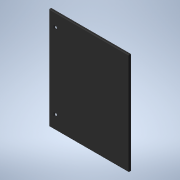
# Autodesk Inventor part: 1676X_01_01(1)_P2
Saved by Autodesk Inventor 2021 (Build 250183000, 183)
## iProperties
Created: 2025-05-05
Part Number: 1676X_01_01(1)_P2
Material: Generic
Catalog Web Link: www.cadenas.de
Description: AE 2.0 Einzeltuer-AE 2.0 Einzeltuer
Vendor: RITTAL
Document SubType Name: Modeling
Designer: psAdmin
Manufacturer: RITTAL
Mass: 1137.32 g
Surface Area: 10932.5 cm^2
Volume: 1137.32 cm^3
Density: 1 g/cm^3
Appearance: PSOLRGB-175-175-175
Category: PARTsolutions
Company: RITTAL
Title: 1676X_01_01(1)_P2
Author: Cadenas PARTsolutions
Comments: AE 2.0 Einzeltuer
PSOL_IDENT_0: {$CADENAS_DATA/23d-libs/rittal/schaltschranksys/kompakt_schaltschr/parts_ae_2_0/einzeltuer_ae_2_0.pr
PSOL_IDENT_1: j},198 {VTYP=3D},{NB=1676X_01_01(1)_P2},{LINA=1676X_01_01(1)_P2},{NN=AE 2.0 Einzeltuer},{DATE=28.04.
PSOL_IDENT_2: 2025 21:11:31},{GEOMDATE=11.04.2025 11:21:47},{VERSION=},{LINEID=330},{WBVAR=DETAIL},{WBNUMERIC=DETA
PSOL_IDENT_3: IL}  {NB=1676X_01_01(1)_P2},{LINA=1676X_01_01(1)_P2},{KT=DUMMY},{BEST=1676X},{DETAIL=1},{BEZ1=Neues
PSOL_IDENT_4: Kompaktgehäuse},{BEZ2=Stahlblech},{BEZ3=eintürig},{B=600},{H=760},{VERS=1},{W=595},{W1=525},{W3=0},{
PSOL_IDENT_5: HH=755},{H1=635},{H2=700},{H4=58.0},{H5=560.000},{H6=600.000},{H7=500.000},{D=15.0},{ST=2.0},{R1=5.0
PSOL_IDENT_6: },{GEW=0},{CNSECLASS51=27-18-01-02},{CNSECLASS70=27-18-01-01},{CNSECLASS80=27-18-01-01},{CNSETIM40=E
PSOL_IDENT_7: C000261}
NB: 1676X_01_01(1)_P2
NN: AE 2.0 Einzeltuer
NT: AE 2.0 Einzeltuer
NBSYN: $BEST._01_01($DETAIL.)_P2
LINA: 1676X_01_01(1)_P2
CATALOG: Rittal
BEST: 1676X
DETAIL: hoch
BEZ1: Neues Kompaktgehäuse
BEZ2: Stahlblech
BEZ3: eintürig
B: 600
H: 760
VERS: 1
W: 595
W1: 525
W3: 0
HH: 755
H1: 635
H2: 700
H4: 58
H5: 560
H6: 600
H7: 500
D: 15
ST: 2
R1: 5
GEW: 0
CNSECLASS70: 27-18-01-01
CNSECLASS80: 27-18-01-01
SUPPLIER: RITTAL
ARTICLENO: 1676X_01_01(1)_P2
BOMINFO: 1676X_01_01(1)_P2
CREATOR: CADENAS GmbH
Autodesk Inventor part; units mm, degrees
sketch "Sketch_1" plane through (0, 0, 0) normal (0, 1, 0) x (1, 0, 0)
  arc A0 (-297.5, 5) -> (-292.5, 0) centre (-292.5, 5) ccw
  line L0 (-292.5, 0) -> (292.5, 0)
  arc A1 (292.5, 0) -> (297.5, 5) centre (292.5, 5) ccw
  line L1 (297.5, 5) -> (297.5, 15)
  line L2 (297.5, 15) -> (295.5, 15)
  line L3 (295.5, 15) -> (295.5, 5)
  arc A2 (292.5, 2) -> (295.5, 5) centre (292.5, 5) ccw
  line L4 (292.5, 2) -> (-292.5, 2)
  arc A3 (-295.5, 5) -> (-292.5, 2) centre (-292.5, 5) ccw
  line L5 (-295.5, 5) -> (-295.5, 15)
  line L6 (-295.5, 15) -> (-297.5, 15)
  line L7 (-297.5, 15) -> (-297.5, 5)
  constraints: 16 end point, 8 point on circle, 4 centre point
extrude "Extrusion1" add sketch "Sketch_1" along normal mid plane 745
sketch "Sketch_3" plane through (0, 372.5, 0) normal (0, 1, 0) x (1, 0, 0)
  line L0 (292.5, 0) -> (292.5, 15)
  arc A0 (292.5, 2) -> (295.5, 5) centre (292.5, 5) ccw
  line L1 (295.5, 5) -> (295.5, 15)
  line L2 (295.5, 15) -> (297.5, 15)
  line L3 (297.5, 15) -> (297.5, 5)
  arc A1 (292.5, 0) -> (297.5, 5) centre (292.5, 5) ccw
  line L4 (292.5, 0) -> (292.5, 2)
  constraints: 10 end point, 4 point on circle, 2 centre point
revolve "Revolution1" add sketch "Sketch_3" angle 90 about axis through (292.5, 372.5, 0) along (0, 0, 1)
sketch "Sketch_4" plane through (0, 372.5, 0) normal (0, 1, 0) x (1, 0, 0)
  line L0 (-292.5, 15) -> (-292.5, 0)
  arc A0 (-297.5, 5) -> (-292.5, 0) centre (-292.5, 5) ccw
  line L1 (-297.5, 5) -> (-297.5, 15)
  line L2 (-297.5, 15) -> (-295.5, 15)
  line L3 (-295.5, 15) -> (-295.5, 5)
  arc A1 (-295.5, 5) -> (-292.5, 2) centre (-292.5, 5) ccw
  line L4 (-292.5, 2) -> (-292.5, 0)
  constraints: 10 end point, 4 point on circle, 2 centre point
revolve "Revolution2" add sketch "Sketch_4" angle 90 about axis through (-292.5, 372.5, -15) along (0, 0, -1)
sketch "Sketch_5" plane through (0, -372.5, 0) normal (0, 1, 0) x (1, 0, 0)
  line L0 (292.5, 0) -> (292.5, 15)
  arc A0 (292.5, 2) -> (295.5, 5) centre (292.5, 5) ccw
  line L1 (295.5, 5) -> (295.5, 15)
  line L2 (295.5, 15) -> (297.5, 15)
  line L3 (297.5, 15) -> (297.5, 5)
  arc A1 (292.5, 0) -> (297.5, 5) centre (292.5, 5) ccw
  line L4 (292.5, 0) -> (292.5, 2)
  constraints: 10 end point, 4 point on circle, 2 centre point
revolve "Revolution3" add sketch "Sketch_5" angle 90 about axis through (292.5, -372.5, 0) along (0, 0, -1)
sketch "Sketch_6" plane through (0, -372.5, 0) normal (0, 1, 0) x (1, 0, 0)
  line L0 (-292.5, 15) -> (-292.5, 0)
  arc A0 (-297.5, 5) -> (-292.5, 0) centre (-292.5, 5) ccw
  line L1 (-297.5, 5) -> (-297.5, 15)
  line L2 (-297.5, 15) -> (-295.5, 15)
  line L3 (-295.5, 15) -> (-295.5, 5)
  arc A1 (-295.5, 5) -> (-292.5, 2) centre (-292.5, 5) ccw
  line L4 (-292.5, 2) -> (-292.5, 0)
  constraints: 10 end point, 4 point on circle, 2 centre point
revolve "Revolution4" add sketch "Sketch_6" angle 90 about axis through (-292.5, -372.5, -15) along (0, 0, 1)
sketch "Sketch_2" plane through (0, 0, 0) normal (1, 0, 0) x (0, 0, -1)
  line L0 (0, 372.5) -> (0, -372.5)
  arc A0 (0, -372.5) -> (5, -377.5) centre (5, -372.5) ccw
  line L1 (5, -377.5) -> (15, -377.5)
  line L2 (15, -377.5) -> (15, -375.5)
  line L3 (15, -375.5) -> (5, -375.5)
  arc A1 (2, -372.5) -> (5, -375.5) centre (5, -372.5) ccw
  line L4 (2, -372.5) -> (2, 372.5)
  arc A2 (5, 375.5) -> (2, 372.5) centre (5, 372.5) ccw
  line L5 (5, 375.5) -> (15, 375.5)
  line L6 (15, 375.5) -> (15, 377.5)
  line L7 (15, 377.5) -> (5, 377.5)
  arc A3 (5, 377.5) -> (0, 372.5) centre (5, 372.5) ccw
  constraints: 16 end point, 8 point on circle, 4 centre point
extrude "Extrusion2" add sketch "Sketch_2" along normal mid plane 585
sketch "Sketch_44" plane through (281, 0, 0) normal (1, 0, 0) x (0, 0, -1)
  line L0 (2, -354.6934) -> (2, 354.6934)
  line L1 (2, 354.6934) -> (8, 354.6934)
  line L2 (8, 354.6934) -> (7.5, 338)
  line L3 (7.5, 338) -> (7.5, -338)
  line L4 (7.5, -338) -> (8, -354.6934)
  line L5 (8, -354.6934) -> (2, -354.6934)
  line L6 (2, -354.6934) -> (2, 354.6934)
  constraints: 14 end point
revolve "Revolution5" add sketch "Sketch_44" angle 180 mid plane about axis through (281, -354.6934, -2) along (0, 1, 0)
sketch "Sketch_45" plane through (0, 354.6934, 0) normal (0, 1, 0) x (1, 0, 0)
  line L0 (291, 8) -> (291, 2)
  line L1 (275, 2) -> (287, 2)
  arc A0 (287, 2) -> (275, 2) centre (281, 2) ccw
  constraints: 4 end point, 2 point on circle, 1 centre point
revolve "Revolution6" add sketch "Sketch_45" angle 39.715 about axis through (291, 354.6934, -8) along (0, 0, -1)
sketch "Sketch_47" plane through (0, 354.6934, 0) normal (0, 1, 0) x (1, 0, 0)
  line L0 (-291, 2) -> (-291, 8)
  line L1 (-287, 2) -> (-275, 2)
  arc A0 (-275, 2) -> (-287, 2) centre (-281, 2) ccw
  constraints: 4 end point, 2 point on circle, 1 centre point
revolve "Revolution7" add sketch "Sketch_47" angle 39.715 about axis through (-291, 354.6934, -2) along (0, 0, 1)
sketch "Sketch_46" plane through (291, 354.6934, 0) normal (-0.6389711, -0.7692308, 0) x (-0.7692308, 0.6389711, 0)
  line L0 (13, 7.1962) -> (13, 2)
  line L1 (13, 2) -> (4, 2)
  arc A0 (13, 7.1962) -> (4, 2) centre (10, 2) ccw
  line L2 (13, 7.1962) -> (13, 2)
  constraints: 6 end point, 2 point on circle, 1 centre point
revolve "Revolution8" add sketch "Sketch_46" angle 169.43 about axis through (281, 363, -7.1962) along (0, 0, 1)
sketch "Sketch_49" plane through (-291, 354.6934, 0) normal (-0.6389711, 0.7692308, 0) x (0.7692308, 0.6389711, 0)
  line L0 (13, 7.1962) -> (13, 2)
  line L1 (13, 2) -> (4, 2)
  arc A0 (13, 7.1962) -> (4, 2) centre (10, 2) ccw
  line L2 (13, 7.1962) -> (13, 2)
  constraints: 6 end point, 2 point on circle, 1 centre point
revolve "Revolution9" add sketch "Sketch_49" angle 169.43 about axis through (-281, 363, -7.1962) along (0, 0, -1)
sketch "Sketch_48" plane through (281, 363, 0) normal (-0.7692308, -0.6389711, 0) x (-0.6389711, 0.7692308, 0)
  line L0 (13, 8) -> (13, 2)
  line L1 (-3, 2) -> (9, 2)
  arc A0 (9, 2) -> (-3, 2) centre (3, 2) ccw
  constraints: 4 end point, 2 point on circle, 1 centre point
revolve "Revolution10" add sketch "Sketch_48" angle 39.715 about axis through (272.6934, 373, -8) along (0, 0, -1)
sketch "Sketch_50" plane through (-281, 363, 0) normal (-0.7692308, 0.6389711, 0) x (0.6389711, 0.7692308, 0)
  line L0 (13, 8) -> (13, 2)
  line L1 (-3, 2) -> (9, 2)
  arc A0 (9, 2) -> (-3, 2) centre (3, 2) ccw
  constraints: 4 end point, 2 point on circle, 1 centre point
revolve "Revolution11" add sketch "Sketch_50" angle 39.715 about axis through (-272.6934, 373, -8) along (0, 0, 1)
sketch "Sketch_51" plane through (-281, 0, 0) normal (1, 0, 0) x (0, 0, -1)
  line L0 (2, -354.6934) -> (2, 354.6934)
  line L1 (2, 354.6934) -> (8, 354.6934)
  line L2 (8, 354.6934) -> (7.5, 338)
  line L3 (7.5, 338) -> (7.5, -338)
  line L4 (7.5, -338) -> (8, -354.6934)
  line L5 (8, -354.6934) -> (2, -354.6934)
  line L6 (2, -354.6934) -> (2, 354.6934)
  constraints: 14 end point
revolve "Revolution12" add sketch "Sketch_51" angle 180 mid plane about axis through (-281, -354.6934, -2) along (0, 1, 0)
sketch "Sketch_52" plane through (0, -354.6934, 0) normal (0, 1, 0) x (1, 0, 0)
  line L0 (291, 8) -> (291, 2)
  line L1 (275, 2) -> (287, 2)
  arc A0 (287, 2) -> (275, 2) centre (281, 2) ccw
  constraints: 4 end point, 2 point on circle, 1 centre point
revolve "Revolution13" add sketch "Sketch_52" angle 39.715 about axis through (291, -354.6934, -8) along (0, 0, 1)
sketch "Sketch_53" plane through (0, -354.6934, 0) normal (0, 1, 0) x (1, 0, 0)
  line L0 (-291, 2) -> (-291, 8)
  line L1 (-287, 2) -> (-275, 2)
  arc A0 (-275, 2) -> (-287, 2) centre (-281, 2) ccw
  constraints: 4 end point, 2 point on circle, 1 centre point
revolve "Revolution14" add sketch "Sketch_53" angle 39.715 about axis through (-291, -354.6934, -2) along (0, 0, -1)
sketch "Sketch_54" plane through (291, -354.6934, 0) normal (0.6389711, -0.7692308, 0) x (-0.7692308, -0.6389711, 0)
  line L0 (13, 7.1962) -> (13, 2)
  line L1 (13, 2) -> (4, 2)
  arc A0 (13, 7.1962) -> (4, 2) centre (10, 2) ccw
  line L2 (13, 7.1962) -> (13, 2)
  constraints: 6 end point, 2 point on circle, 1 centre point
revolve "Revolution15" add sketch "Sketch_54" angle 169.43 about axis through (281, -363, -7.1962) along (0, 0, -1)
sketch "Sketch_55" plane through (281, -363, 0) normal (0.7692308, -0.6389711, 0) x (-0.6389711, -0.7692308, 0)
  line L0 (13, 8) -> (13, 2)
  line L1 (-3, 2) -> (9, 2)
  arc A0 (9, 2) -> (-3, 2) centre (3, 2) ccw
  constraints: 4 end point, 2 point on circle, 1 centre point
revolve "Revolution16" add sketch "Sketch_55" angle 39.715 about axis through (272.6934, -373, -8) along (0, 0, 1)
sketch "Sketch_56" plane through (-291, -354.6934, 0) normal (-0.6389711, -0.7692308, 0) x (-0.7692308, 0.6389711, 0)
  line L0 (-13, 2) -> (-13, 7.1962)
  arc A0 (-4, 2) -> (-13, 7.1962) centre (-10, 2) ccw
  line L1 (-4, 2) -> (-13, 2)
  line L2 (-13, 2) -> (-13, 7.1962)
  constraints: 6 end point, 2 point on circle, 1 centre point
revolve "Revolution17" add sketch "Sketch_56" angle 169.43 about axis through (-281, -363, -2) along (0, 0, 1)
sketch "Sketch_57" plane through (-281, -363, 0) normal (0.7692308, 0.6389711, 0) x (0.6389711, -0.7692308, 0)
  line L0 (13, 8) -> (13, 2)
  line L1 (-3, 2) -> (9, 2)
  arc A0 (9, 2) -> (-3, 2) centre (3, 2) ccw
  constraints: 4 end point, 2 point on circle, 1 centre point
revolve "Revolution18" add sketch "Sketch_57" angle 39.715 about axis through (-272.6934, -373, -8) along (0, 0, -1)
sketch "Sketch_58" plane through (0, 363, 0) normal (0, 1, 0) x (1, 0, 0)
  line L0 (272.6934, 2) -> (-272.6934, 2)
  line L1 (-272.6934, 2) -> (-272.6934, 8)
  line L2 (-272.6934, 8) -> (272.6934, 8)
  line L3 (272.6934, 8) -> (272.6934, 2)
  line L4 (272.6934, 2) -> (-272.6934, 2)
  constraints: 10 end point
revolve "Revolution19" add sketch "Sketch_58" angle 180 mid plane about axis through (272.6934, 363, -2) along (-1, 0, 0)
sketch "Sketch_59" plane through (0, -363, 0) normal (0, 1, 0) x (1, 0, 0)
  line L0 (272.6934, 2) -> (-272.6934, 2)
  line L1 (-272.6934, 2) -> (-272.6934, 8)
  line L2 (-272.6934, 8) -> (272.6934, 8)
  line L3 (272.6934, 8) -> (272.6934, 2)
  line L4 (272.6934, 2) -> (-272.6934, 2)
  constraints: 10 end point
revolve "Revolution20" add sketch "Sketch_59" angle 180 mid plane about axis through (272.6934, -363, -2) along (-1, 0, 0)
sketch "Sketch_7" plane through (0, -317.5, 0) normal (0, 1, 0) x (1, 0, 0)
  arc A0 (290.5, 15.1) -> (290.5, 6.9) centre (290.5, 11) ccw
  line L0 (290.5, 6.9) -> (295.5, 6.9)
  line L1 (295.5, 6.9) -> (295.5, 8.4)
  line L2 (295.5, 8.4) -> (290.5, 8.4)
  arc A1 (290.5, 13.6) -> (290.5, 8.4) centre (290.5, 11) ccw
  line L3 (290.5, 13.6) -> (295.5, 13.6)
  line L4 (295.5, 13.6) -> (295.5, 15.1)
  line L5 (295.5, 15.1) -> (290.5, 15.1)
  constraints: 12 end point, 4 point on circle, 2 centre point
extrude "Extrusion3" add sketch "Sketch_7" along normal mid plane 19.7
sketch "Sketch_8" plane through (0, 317.5, 0) normal (0, 1, 0) x (1, 0, 0)
  arc A0 (290.5, 15.1) -> (290.5, 6.9) centre (290.5, 11) ccw
  line L0 (290.5, 6.9) -> (295.5, 6.9)
  line L1 (295.5, 6.9) -> (295.5, 8.4)
  line L2 (295.5, 8.4) -> (290.5, 8.4)
  arc A1 (290.5, 13.6) -> (290.5, 8.4) centre (290.5, 11) ccw
  line L3 (290.5, 13.6) -> (295.5, 13.6)
  line L4 (295.5, 13.6) -> (295.5, 15.1)
  line L5 (295.5, 15.1) -> (290.5, 15.1)
  constraints: 12 end point, 4 point on circle, 2 centre point
extrude "Extrusion4" add sketch "Sketch_8" along normal mid plane 19.7
sketch "Sketch_11" plane through (0, 0, 0) normal (0, 1, 0) x (1, 0, 0)
  line L0 (254.5, 15.9) -> (254.5, 2)
  line L1 (254.5, 2) -> (255.3, 2)
  line L2 (255.3, 2) -> (255.3, 15.9)
  arc A0 (256.1, 16.7) -> (255.3, 15.9) centre (256.1, 15.9) ccw
  line L3 (256.1, 16.7) -> (268.4, 16.7)
  arc A1 (269.2, 15.9) -> (268.4, 16.7) centre (268.4, 15.9) ccw
  line L4 (269.2, 15.9) -> (269.2, 2)
  line L5 (269.2, 2) -> (270, 2)
  line L6 (270, 2) -> (270, 15.9)
  arc A2 (270, 15.9) -> (268.4, 17.5) centre (268.4, 15.9) ccw
  line L7 (268.4, 17.5) -> (256.1, 17.5)
  arc A3 (256.1, 17.5) -> (254.5, 15.9) centre (256.1, 15.9) ccw
  constraints: 16 end point, 8 point on circle, 4 centre point
extrude "Extrusion5" add sketch "Sketch_11" along normal mid plane 700
sketch "Sketch_12" plane through (0, 0, 0) normal (0, 1, 0) x (1, 0, 0)
  line L0 (-270.5, 15.9) -> (-270.5, 2)
  line L1 (-270.5, 2) -> (-269.7, 2)
  line L2 (-269.7, 2) -> (-269.7, 15.9)
  arc A0 (-268.9, 16.7) -> (-269.7, 15.9) centre (-268.9, 15.9) ccw
  line L3 (-268.9, 16.7) -> (-256.6, 16.7)
  arc A1 (-255.8, 15.9) -> (-256.6, 16.7) centre (-256.6, 15.9) ccw
  line L4 (-255.8, 15.9) -> (-255.8, 2)
  line L5 (-255.8, 2) -> (-255, 2)
  line L6 (-255, 2) -> (-255, 15.9)
  arc A2 (-255, 15.9) -> (-256.6, 17.5) centre (-256.6, 15.9) ccw
  line L7 (-256.6, 17.5) -> (-268.9, 17.5)
  arc A3 (-268.9, 17.5) -> (-270.5, 15.9) centre (-268.9, 15.9) ccw
  constraints: 16 end point, 8 point on circle, 4 centre point
extrude "Extrusion6" add sketch "Sketch_12" along normal mid plane 700
sketch "Sketch_13" plane through (262.25, 0, 0) normal (1, 0, 0) x (0, 0, -1)
  line L0 (14.5, 331) -> (14.5, 320.5)
  arc A0 (14.5, 320.5) -> (15.5, 319.5) centre (15.5, 320.5) ccw
  line L1 (15.5, 319.5) -> (18.5, 319.5)
  line L2 (18.5, 319.5) -> (18.5, -319.5)
  line L3 (18.5, -319.5) -> (15.5, -319.5)
  arc A1 (15.5, -319.5) -> (14.5, -320.5) centre (15.5, -320.5) ccw
  line L4 (14.5, -320.5) -> (14.5, -331)
  arc A2 (14.5, -331) -> (15.5, -332) centre (15.5, -331) ccw
  line L5 (15.5, -332) -> (22.5, -332)
  line L6 (22.5, -332) -> (22.5, 332)
  line L7 (22.5, 332) -> (15.5, 332)
  arc A3 (15.5, 332) -> (14.5, 331) centre (15.5, 331) ccw
  constraints: 16 end point, 8 point on circle, 4 centre point
extrude "Extrusion7" cut sketch "Sketch_13" along normal mid plane 15.5
sketch "Sketch_15" plane through (262.25, 0, 0) normal (1, 0, 0) x (0, 0, -1)
  line L0 (15.5, 300) -> (17.5, 300)
  line L1 (17.5, 300) -> (17.5, 296.5)
  line L2 (17.5, 296.5) -> (16.7, 296.5)
  line L3 (16.7, 296.5) -> (16.7, 296.7)
  arc A0 (16.7, 296.7) -> (16.45, 296.95) centre (16.45, 296.7) ccw
  line L4 (16.45, 296.95) -> (15.5, 296.95)
  line L5 (15.5, 296.95) -> (15.5, 300)
  line L6 (15.5, 300) -> (17.5, 300)
  constraints: 14 end point, 2 point on circle, 1 centre point
revolve "Revolution21" add sketch "Sketch_15" angle 360 about axis through (262.25, 300, -15.5) along (0, 0, 1)
sketch "Sketch_14" plane through (-262.75, 0, 0) normal (1, 0, 0) x (0, 0, -1)
  line L0 (14.5, 331) -> (14.5, 320.5)
  arc A0 (14.5, 320.5) -> (15.5, 319.5) centre (15.5, 320.5) ccw
  line L1 (15.5, 319.5) -> (18.5, 319.5)
  line L2 (18.5, 319.5) -> (18.5, -319.5)
  line L3 (18.5, -319.5) -> (15.5, -319.5)
  arc A1 (15.5, -319.5) -> (14.5, -320.5) centre (15.5, -320.5) ccw
  line L4 (14.5, -320.5) -> (14.5, -331)
  arc A2 (14.5, -331) -> (15.5, -332) centre (15.5, -331) ccw
  line L5 (15.5, -332) -> (22.5, -332)
  line L6 (22.5, -332) -> (22.5, 332)
  line L7 (22.5, 332) -> (15.5, 332)
  arc A3 (15.5, 332) -> (14.5, 331) centre (15.5, 331) ccw
  constraints: 16 end point, 8 point on circle, 4 centre point
extrude "Extrusion8" cut sketch "Sketch_14" along normal mid plane 15.5
pattern_linear "Rectangular Pattern1" count 25 spacing 25 along (0, -1, 0) of "Revolution21"
sketch "Sketch_17" plane through (262.25, 0, 0) normal (1, 0, 0) x (0, 0, -1)
  line L0 (15.5, 300) -> (18, 300)
  line L1 (18, 300) -> (18, 297)
  line L2 (18, 297) -> (17.5, 297)
  line L3 (17.5, 297) -> (17.5, 297.25)
  arc A0 (17.5, 297.25) -> (17, 297.75) centre (17, 297.25) ccw
  line L4 (17, 297.75) -> (15.5, 297.75)
  line L5 (15.5, 297.75) -> (15.5, 300)
  line L6 (15.5, 300) -> (18, 300)
  constraints: 14 end point, 2 point on circle, 1 centre point
revolve "Revolution22" cut sketch "Sketch_17" angle 360 about axis through (262.25, 300, -15.5) along (0, 0, 1)
pattern_linear "Rectangular Pattern2" count 25 spacing 25 along (0, -1, 0) of "Revolution22"
sketch "Sketch_19" plane through (-262.75, 0, 0) normal (1, 0, 0) x (0, 0, -1)
  line L0 (15.5, 250) -> (17.5, 250)
  line L1 (17.5, 250) -> (17.5, 246.5)
  line L2 (17.5, 246.5) -> (16.7, 246.5)
  line L3 (16.7, 246.5) -> (16.7, 246.7)
  arc A0 (16.7, 246.7) -> (16.45, 246.95) centre (16.45, 246.7) ccw
  line L4 (16.45, 246.95) -> (15.5, 246.95)
  line L5 (15.5, 246.95) -> (15.5, 250)
  line L6 (15.5, 250) -> (17.5, 250)
  constraints: 14 end point, 2 point on circle, 1 centre point
revolve "Revolution23" add sketch "Sketch_19" angle 360 about axis through (-262.75, 250, -15.5) along (0, 0, 1)
pattern_linear "Rectangular Pattern3" count 21 spacing 25 along (0, -1, 0) of "Revolution23"
sketch "Sketch_21" plane through (-262.75, 0, 0) normal (1, 0, 0) x (0, 0, -1)
  line L0 (15.5, 250) -> (18, 250)
  line L1 (18, 250) -> (18, 247)
  line L2 (18, 247) -> (17.5, 247)
  line L3 (17.5, 247) -> (17.5, 247.25)
  arc A0 (17.5, 247.25) -> (17, 247.75) centre (17, 247.25) ccw
  line L4 (17, 247.75) -> (15.5, 247.75)
  line L5 (15.5, 247.75) -> (15.5, 250)
  line L6 (15.5, 250) -> (18, 250)
  constraints: 14 end point, 2 point on circle, 1 centre point
revolve "Revolution24" cut sketch "Sketch_21" angle 360 about axis through (-262.75, 250, -15.5) along (0, 0, 1)
pattern_linear "Rectangular Pattern4" count 21 spacing 25 along (0, -1, 0) of "Revolution24"
sketch "Sketch_23" plane through (0, 0, -17.5) normal (0, 0, 1) x (1, 0, 0)
  line L0 (260.25, 281.25) -> (264.25, 281.25)
  line L1 (264.25, 281.25) -> (264.25, 293.75)
  line L2 (264.25, 293.75) -> (260.25, 293.75)
  line L3 (260.25, 293.75) -> (260.25, 281.25)
  constraints: 8 end point
extrude "Extrusion9" cut sketch "Sketch_23" along normal blind 0.8
pattern_linear "Rectangular Pattern5" count 24 spacing 25 along (0, -1, 0) of "Extrusion9"
sketch "Sketch_25" plane through (0, 0, -17.5) normal (0, 0, 1) x (1, 0, 0)
  line L0 (-264.75, 231.25) -> (-260.75, 231.25)
  line L1 (-260.75, 231.25) -> (-260.75, 243.75)
  line L2 (-260.75, 243.75) -> (-264.75, 243.75)
  line L3 (-264.75, 243.75) -> (-264.75, 231.25)
  constraints: 8 end point
extrude "Extrusion10" cut sketch "Sketch_25" along normal blind 0.8
pattern_linear "Rectangular Pattern6" count 20 spacing 25 along (0, -1, 0) of "Extrusion10"
sketch "Sketch_27" plane through (0, 0, -17.5) normal (0, 0, 1) x (1, 0, 0)
  line L0 (-265.6, 297) -> (-265.6, 263)
  arc A0 (-265.6, 263) -> (-262.6, 260) centre (-262.6, 263) ccw
  line L1 (-262.6, 260) -> (-250.6, 260)
  line L2 (-250.6, 260) -> (-250.6, 300)
  line L3 (-250.6, 300) -> (-262.6, 300)
  arc A1 (-262.6, 300) -> (-265.6, 297) centre (-262.6, 297) ccw
  constraints: 8 end point, 4 point on circle, 2 centre point
extrude "Extrusion11" cut sketch "Sketch_27" along normal blind 15.5
sketch "Sketch_28" plane through (0, 0, -17.5) normal (0, 0, 1) x (1, 0, 0)
  line L0 (-265.6, -263) -> (-265.6, -297)
  arc A0 (-265.6, -297) -> (-262.6, -300) centre (-262.6, -297) ccw
  line L1 (-262.6, -300) -> (-250.6, -300)
  line L2 (-250.6, -300) -> (-250.6, -260)
  line L3 (-250.6, -260) -> (-262.6, -260)
  arc A1 (-262.6, -260) -> (-265.6, -263) centre (-262.6, -263) ccw
  constraints: 8 end point, 4 point on circle, 2 centre point
extrude "Extrusion12" cut sketch "Sketch_28" along normal blind 15.5
sketch "Sketch_29" plane through (0, 0, -17.5) normal (0, 0, 1) x (1, 0, 0)
  line L0 (257, 332) -> (257, 331)
  line L1 (257, 331) -> (267.5, 331)
  line L2 (267.5, 331) -> (267.5, 332)
  arc A0 (266.5, 333) -> (267.5, 332) centre (267.5, 333) ccw
  line L3 (266.5, 333) -> (266.5, 340.5)
  arc A1 (266.5, 340.5) -> (258, 340.5) centre (262.25, 340.5) ccw
  line L4 (258, 340.5) -> (258, 333)
  arc A2 (257, 332) -> (258, 333) centre (257, 333) ccw
  constraints: 10 end point, 6 point on circle, 3 centre point
extrude "Extrusion13" cut sketch "Sketch_29" along normal blind 0.8
sketch "Sketch_30" plane through (0, 0, -17.5) normal (0, 0, 1) x (1, 0, 0)
  arc A0 (258, -333) -> (257, -332) centre (257, -333) ccw
  line L0 (258, -333) -> (258, -340.5)
  arc A1 (258, -340.5) -> (266.5, -340.5) centre (262.25, -340.5) ccw
  line L1 (266.5, -340.5) -> (266.5, -333)
  arc A2 (267.5, -332) -> (266.5, -333) centre (267.5, -333) ccw
  line L2 (267.5, -332) -> (267.5, -331)
  line L3 (267.5, -331) -> (257, -331)
  line L4 (257, -331) -> (257, -332)
  constraints: 10 end point, 6 point on circle, 3 centre point
extrude "Extrusion14" cut sketch "Sketch_30" along normal blind 0.8
sketch "Sketch_31" plane through (0, 0, -17.5) normal (0, 0, 1) x (1, 0, 0)
  line L0 (-268, 332) -> (-268, 331)
  line L1 (-268, 331) -> (-257.5, 331)
  line L2 (-257.5, 331) -> (-257.5, 332)
  arc A0 (-258.5, 333) -> (-257.5, 332) centre (-257.5, 333) ccw
  line L3 (-258.5, 333) -> (-258.5, 340.5)
  arc A1 (-258.5, 340.5) -> (-267, 340.5) centre (-262.75, 340.5) ccw
  line L4 (-267, 340.5) -> (-267, 333)
  arc A2 (-268, 332) -> (-267, 333) centre (-268, 333) ccw
  constraints: 10 end point, 6 point on circle, 3 centre point
extrude "Extrusion15" cut sketch "Sketch_31" along normal blind 0.8
sketch "Sketch_32" plane through (0, 0, -17.5) normal (0, 0, 1) x (1, 0, 0)
  arc A0 (-267, -333) -> (-268, -332) centre (-268, -333) ccw
  line L0 (-267, -333) -> (-267, -340.5)
  arc A1 (-267, -340.5) -> (-258.5, -340.5) centre (-262.75, -340.5) ccw
  line L1 (-258.5, -340.5) -> (-258.5, -333)
  arc A2 (-257.5, -332) -> (-258.5, -333) centre (-257.5, -333) ccw
  line L2 (-257.5, -332) -> (-257.5, -331)
  line L3 (-257.5, -331) -> (-268, -331)
  line L4 (-268, -331) -> (-268, -332)
  constraints: 10 end point, 6 point on circle, 3 centre point
extrude "Extrusion16" cut sketch "Sketch_32" along normal blind 0.8
sketch "Sketch_33" plane through (0, 0, 0) normal (0, 0, 1) x (1, 0, 0)
  line L0 (-261.15, 290.65) -> (-261.15, 269.35)
  arc A0 (-261.15, 269.35) -> (-260.65, 268.85) centre (-260.65, 269.35) ccw
  line L1 (-260.65, 268.85) -> (-239.35, 268.85)
  arc A1 (-239.35, 268.85) -> (-238.85, 269.35) centre (-239.35, 269.35) ccw
  line L2 (-238.85, 269.35) -> (-238.85, 290.65)
  arc A2 (-238.85, 290.65) -> (-239.35, 291.15) centre (-239.35, 290.65) ccw
  line L3 (-239.35, 291.15) -> (-252.65, 291.15)
  arc A3 (-253.15, 291.65) -> (-252.65, 291.15) centre (-252.65, 291.65) ccw
  line L4 (-253.15, 291.65) -> (-253.15, 292.15)
  arc A4 (-253.15, 292.15) -> (-253.65, 292.65) centre (-253.65, 292.15) ccw
  line L5 (-253.65, 292.65) -> (-258.65, 292.65)
  arc A5 (-258.65, 292.65) -> (-259.15, 292.15) centre (-258.65, 292.15) ccw
  line L6 (-259.15, 292.15) -> (-259.15, 291.65)
  arc A6 (-259.65, 291.15) -> (-259.15, 291.65) centre (-259.65, 291.65) ccw
  line L7 (-259.65, 291.15) -> (-260.65, 291.15)
  arc A7 (-260.65, 291.15) -> (-261.15, 290.65) centre (-260.65, 290.65) ccw
  constraints: 16 end point, 16 point on circle, 8 centre point
extrude "Extrusion17" cut sketch "Sketch_33" against normal blind 2
sketch "Sketch_34" plane through (0, 0, 0) normal (0, 0, 1) x (1, 0, 0)
  line L0 (-261.15, -269.35) -> (-261.15, -290.65)
  arc A0 (-261.15, -290.65) -> (-260.65, -291.15) centre (-260.65, -290.65) ccw
  line L1 (-260.65, -291.15) -> (-239.35, -291.15)
  arc A1 (-239.35, -291.15) -> (-238.85, -290.65) centre (-239.35, -290.65) ccw
  line L2 (-238.85, -290.65) -> (-238.85, -269.35)
  arc A2 (-238.85, -269.35) -> (-239.35, -268.85) centre (-239.35, -269.35) ccw
  line L3 (-239.35, -268.85) -> (-252.65, -268.85)
  arc A3 (-253.15, -268.35) -> (-252.65, -268.85) centre (-252.65, -268.35) ccw
  line L4 (-253.15, -268.35) -> (-253.15, -267.85)
  arc A4 (-253.15, -267.85) -> (-253.65, -267.35) centre (-253.65, -267.85) ccw
  line L5 (-253.65, -267.35) -> (-258.65, -267.35)
  arc A5 (-258.65, -267.35) -> (-259.15, -267.85) centre (-258.65, -267.85) ccw
  line L6 (-259.15, -267.85) -> (-259.15, -268.35)
  arc A6 (-259.65, -268.85) -> (-259.15, -268.35) centre (-259.65, -268.35) ccw
  line L7 (-259.65, -268.85) -> (-260.65, -268.85)
  arc A7 (-260.65, -268.85) -> (-261.15, -269.35) centre (-260.65, -269.35) ccw
  constraints: 16 end point, 16 point on circle, 8 centre point
extrude "Extrusion18" cut sketch "Sketch_34" against normal blind 2
ref_plane "ET_XY" through (290.5, -317.5, -11) normal (0, 1, 0) x (1, 0, 0)
ref_plane "ET_YZ" through (290.5, -317.5, -11) normal (1, 0, 0) x (0, 0, -1)
ref_plane "ET_ZX" through (290.5, -317.5, -11) normal (0, 0, -1) x (0, 1, 0)
ref_plane "SC_XY" through (295.5, 0, 0) normal (0, 0, -1) x (1, 0, 0)
ref_plane "SC_YZ" through (295.5, 0, 0) normal (1, 0, 0) x (0, -1, 0)
ref_plane "SC_ZX" through (295.5, 0, 0) normal (0, -1, 0) x (0, 0, -1)
ref_plane "VV1_XY" through (-250, 280, 0) normal (0, 0, -1) x (1, 0, 0)
ref_plane "VV1_YZ" through (-250, 280, 0) normal (1, 0, 0) x (0, -1, 0)
ref_plane "VV1_ZX" through (-250, 280, 0) normal (0, -1, 0) x (0, 0, -1)
ref_plane "VV2_XY" through (-250, -280, 0) normal (0, 0, -1) x (1, 0, 0)
ref_plane "VV2_YZ" through (-250, -280, 0) normal (1, 0, 0) x (0, -1, 0)
ref_plane "VV2_ZX" through (-250, -280, 0) normal (0, -1, 0) x (0, 0, -1)
ref_plane "to_Auflaufelement_XY" through (-262.75, -340.5, -17.5) normal (0, 0, 1) x (1, 0, 0)
ref_plane "to_Auflaufelement_YZ" through (-262.75, -340.5, -17.5) normal (1, 0, 0) x (0, 1, 0)
ref_plane "to_Auflaufelement_ZX" through (-262.75, -340.5, -17.5) normal (0, 1, 0) x (0, 0, 1)
body "Solid1"
